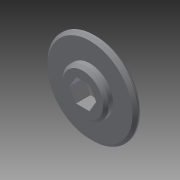
# Autodesk Inventor part: Sprocket Large
Saved by Autodesk Inventor 2015 (Build 190159000, 159)
## iProperties
Created: 2015-01-11
Part Number: Sprocket Large
Material: Generic
Document SubType Name: Modeling
Designer: chapale16
Density: 1 g/cm^3
Appearance: Default
Author: chapale16
Autodesk Inventor part; units mm, degrees
ref_plane "YZ Plane" through (0, 0, 0) normal (1, 0, 0) x (0, 1, 0)
ref_plane "XZ Plane" through (0, 0, 0) normal (0, 1, 0) x (-1, 0, 0)
ref_plane "XY Plane" through (0, 0, 0) normal (0, 0, 1) x (1, 0, 0)
sketch "Sketch1" plane through (0, 0, 0) normal (0, 0, 1) x (1, 0, 0)
  circle A0 centre (0, 0) radius 24.9555
  line L0 (3.7176, 6.32) -> (7.3321, -0.0596)
  line L1 (7.3321, -0.0596) -> (3.6145, -6.3796)
  line L2 (3.6145, -6.3796) -> (-3.7176, -6.32)
  line L3 (-3.7176, -6.32) -> (-7.3321, 0.0596)
  line L4 (-7.3321, 0.0596) -> (-3.6145, 6.3796)
  line L5 (-3.6145, 6.3796) -> (3.7176, 6.32)
  dimension "d0" = 49.911
  dimension "d14" = 6.35
  constraints: 12 end point, 2 coincident, 1 centre point, 13 other
  measures "d0" diameter of A0
  measures "d14" distance from line of L5 A0.centre
extrude "Extrusion3" add sketch "Sketch1" along normal blind 3.937
chamfer "Chamfer3" distance 1.524 angle 45 1 edges at (-24.9555, 0, 3.937)
chamfer "Chamfer4" distance 1.524 angle 45 1 edges at (-24.9555, 0, 0)
sketch "Sketch4" plane through (0, 0, 3.937) normal (0, 0, 1) x (1, 0, 0)
  circle A0 centre (0, 0) radius 23.4315 projected
  line L0 (3.7176, 6.32) -> (7.3321, -0.0596)
  line L1 (7.3321, -0.0596) -> (3.6145, -6.3796)
  line L2 (3.6145, -6.3796) -> (-3.7176, -6.32)
  line L3 (-3.7176, -6.32) -> (-7.3321, 0.0596)
  line L4 (-7.3321, 0.0596) -> (-3.6145, 6.3796)
  line L5 (-3.6145, 6.3796) -> (3.7176, 6.32)
  circle A1 centre (0, 0) radius 12.7
  dimension "d23" = 25.4
  constraints: 12 end point, 2 coincident, 1 centre point, 13 other
  measures "d23" diameter of A1
extrude "Extrusion4" add sketch "Sketch4" along normal blind 3.937 contours A1
chamfer "Chamfer5" distance 1.524 angle 45 1 edges at (-12.7, 0, 7.874)
body "Solid2"
